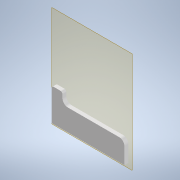
# Autodesk Inventor part: bracera
Saved by Autodesk Inventor 2021 (Build 250183000, 183)
## iProperties
Created: 2021-03-18
Part Number: bracera
Material: Generic
Document SubType Name: Modeling
Designer: andre
Density: 1 g/cm^3
Appearance: Default
Author: andre
Autodesk Inventor part; units mm, degrees
ref_plane "YZ Plane" through (0, 0, 0) normal (1, 0, 0) x (0, 1, 0)
ref_plane "XZ Plane" through (0, 0, 0) normal (0, 1, 0) x (-1, 0, 0)
ref_plane "XY Plane" through (0, 0, 0) normal (0, 0, 1) x (1, 0, 0)
ref_plane "Work Plane1" through (0, 0, 0) normal (0, 0, 1) x (1, 0, 0)
sketch "Sketch1" plane through (0, 0, 0) normal (0, 0, 1) x (1, 0, 0)
  line L0 (0, 0) -> (675, 0) projected
  line L1 (675, 0) -> (675, 150) projected
  line L2 (100, 150) -> (675, 150) projected
  line L3 (100, 150) -> (100, 850) projected
  line L4 (0, 850) -> (100, 850) projected
  line L5 (0, 0) -> (0, 850) projected
  line L6 (0, 0) -> (100, 0)
  line L7 (80, 300) -> (20, 300)
  line L8 (0, 280) -> (0, 0)
  line L9 (100, 0) -> (675, 0)
  line L10 (675, 0) -> (675, 150)
  line L11 (625, 200) -> (150, 200)
  line L12 (100, 200) -> (100, 0)
  line L13 (100, 0) -> (100, 150)
  line L14 (100, 250) -> (100, 280)
  arc A0 (100, 280) -> (80, 300) centre (80, 280) ccw
  arc A1 (20, 300) -> (0, 280) centre (20, 280) ccw
  arc A2 (675, 150) -> (625, 200) centre (625, 150) ccw
  arc A3 (100, 250) -> (150, 200) centre (150, 250) ccw
  point P0 (100, 300)
  point P1 (0, 300)
  point P2 (675, 200)
  dimension "d0" = 150
  dimension "d1" = 200
  dimension "d2" = 300
  dimension "d3" = 20
  dimension "d4" = 20
  dimension "d5" = 50
  constraints: 19 end point, 9 point on line, 8 point on circle, 8 tangent, 5 parallel, 4 centre point, 3 perpendicular, 2 horizontal, 1 equal radius
  measures "d0" distance of L0.end L1.end
  measures "d1" distance of L9.end point (675, 200)
  measures "d2" distance of point (0, 300) L0.start
  measures "d3" radius of A0
  measures "d4" radius of A1
  measures "d5" radius of A2
extrude "Extrusion1" add sketch "Sketch1" along normal blind 36 contours L5 A1 L7 A0 L3 L12 L0 | L12 L2 L1 L0 | L3 A3 L11 A2 L2
body "Solid1"
